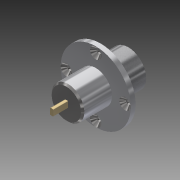
# Autodesk Inventor part: Motor
Saved by Autodesk Inventor 2014 SP1 (Build 180222100, 222)
## iProperties
Created: 2015-03-16
Part Number: Motor
Material: Titanium
Document SubType Name: Modeling
Designer: david
Density: 4.51 g/cm^3
Appearance: Steel - Polished
Mass: 73.2599 g
Surface Area: 59.6795 cm^2
Volume: 16.2439 cm^3
Motor_WheelInterface_Diameter: 30,000 mm
Motor_WheelInterface_Length: 27,000 mm
Motor_FasteningHole_DistanceToCenter: 18,000 mm
Author: david
Autodesk Inventor part; units mm, degrees
ref_plane "YZ Plane" through (0, 0, 0) normal (1, 0, 0) x (0, 1, 0)
ref_plane "XZ Plane" through (0, 0, 0) normal (0, 1, 0) x (-1, 0, 0)
ref_plane "XY Plane" through (0, 0, 0) normal (0, 0, 1) x (1, 0, 0)
sketch "BodySketch" plane through (0, 0, 0) normal (1, 0, 0) x (0, 1, 0)
  line L0 (11, -17) -> (0, -17)
  line L1 (0, -17) -> (0, 21)
  line L2 (0, 25.0354) -> (0, 0) construction
  line L3 (10, 3) -> (21.5, 3)
  line L4 (21.5, 3) -> (21.5, 0)
  line L5 (21.5, 0) -> (11.5, 0)
  line L6 (11.5, -5) -> (9, -5)
  line L7 (9, -5) -> (9, -7)
  line L8 (9, -7) -> (11, -7)
  line L9 (10, 21) -> (10, 3)
  line L10 (11.5, 0) -> (11.5, -5)
  line L11 (11, -7) -> (11, -17)
  line L12 (0, 0) -> (51.0902, 0) construction
  line L13 (10, 21) -> (0, 21)
  dimension "d19" = 10
  dimension "d20" = 21.5
  dimension "d21" = 11.5
  dimension "d22" = 2
  dimension "d23" = 3
  dimension "d24" = 2
  dimension "d26" = 5
  dimension "d37" = 10
  dimension "d39" = 11
  dimension "d40" = 18
  constraints: 28 end point, 3 collinear, 3 horizontal, 3 perpendicular, 2 parallel
  measures "d19" distance between parallel lines of L1 L9
  measures "d20" distance between parallel lines of L1 L4
  measures "d21" distance between parallel lines of L1 L10
  measures "d22" distance between parallel lines of L11 L7
  measures "d23" distance between parallel lines of L5 L3
  measures "d24" distance between parallel lines of L8 L6
  measures "d26" distance of L5.end L6.start
  measures "d37" distance between parallel lines of L0 L8
  measures "d39" distance between parallel lines of L1 L11
  measures "d40" distance of L9.start L3.start
revolve "Body" add sketch "BodySketch" angle 360 about axis through (0, 0, 25.0354) along (0, 0, -1)
sketch "FasteningHoleSketch" plane through (0, 0, 0) normal (0, 0, -1) x (-1, 0, 0)
  circle A0 centre (0, 0) radius 11.5 projected
  circle A1 centre (0, 0) radius 21.5 projected
  circle A2 centre (0, 18) radius 1.5
  line L0 (0, 0) -> (0, 24.6979) construction
  circle A3 centre (18, 0) radius 1.5
  circle A4 centre (0, -18) radius 1.5
  circle A5 centre (-18, 0) radius 1.5
  dimension "Motor_FasteningHole_Size" = 3
  dimension "Motor_FasteningHole_DistanceToBorder" = 2
  dimension "d32" = 360
  constraints: 4 centre point, 2 end point, 1 point on line, 1 vertical, 9 other
  measures "Motor_FasteningHole_Size" diameter of A2
extrude "FasteningHole" cut sketch "FasteningHoleSketch" against normal up to surface (3 mm away) contours A2 | A3 | A4 | A5
chamfer "Chamfer1" distance 1 angle 45 1 edges at (0, -10, 21)
chamfer "Chamfer2" distance 2 angle 45 4 edges at (1.5, 18, 3) (19.5, 0, 3) (-16.5, 0, 3) (1.5, -18, 3)
sketch "Sketch4" plane through (0, 0, 21) normal (0, 0, 1) x (1, 0, 0)
  circle A0 centre (0, 0) radius 9 projected
  line L0 (1, 1.7321) -> (1, -1.7321)
  line L1 (-1, 1.7321) -> (-1, -1.7321)
  arc A1 (1, 1.7321) -> (-1, 1.7321) centre (0, 0) ccw
  arc A2 (-1, -1.7321) -> (1, -1.7321) centre (0, 0) ccw
  dimension "d48" = 2
  dimension "d49" = 2
  dimension "d50" = 2
  constraints: 4 end point, 4 point on circle, 2 centre point, 1 coincident, 1 parallel
  measures "d48" distance between parallel lines of L0 L1
  measures "d49" radius of A1
  measures "d50" radius of A2
extrude "Extrusion3" add sketch "Sketch4" along normal blind 9 separate body contours L0 A2 L1 A1
equation "\"Motor_WheelInterface_Diameter\" = 30"
equation "\"Motor_WheelInterface_Length\" = 27"
equation "\"Motor_FasteningHole_DistanceToCenter\" = 18"
